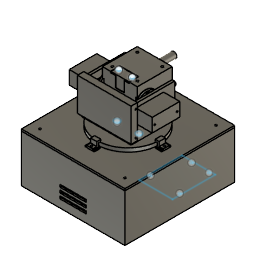
carro_armato_assieme_completo_modificabile_v5_cinematica_stepper_servo_M2_5 (Autodesk Fusion 360 design; units mm, degrees)
part number: 2026-07-14-04-41-23-405
part number: 2026-07-14-04-41-23-631
part number: 2026-07-14-04-41-23-666
part number: 2026-07-14-04-41-25-878
part number: 2026-07-14-04-41-28-136
part number: 2026-07-14-04-41-28-298
part number: 2026-07-14-04-41-30-257
part number: 2026-07-14-04-41-52-420
part number: 2026-07-14-04-41-53-406
part number: 2026-07-14-04-41-55-252
part number: 2026-07-14-04-41-56-766
part number: 2026-07-14-04-42-07-757
part number: 2026-07-14-04-42-11-829
part number: 2026-07-14-04-42-16-180
part number: 2026-07-14-04-42-20-616
part number: 2026-07-14-04-42-24-632
part number: 2026-07-14-04-43-20-199
part number: 2026-07-14-04-43-28-088
part number: 2026-07-14-04-43-36-335
part number: 2026-07-14-04-44-01-058
part number: 2026-07-14-04-44-07-569
part number: 2026-07-14-04-44-14-384
part number: 2026-07-14-04-44-23-421
part number: 2026-07-14-04-44-35-084
part number: 2026-07-14-04-44-58-859
part number: 2026-07-14-04-45-33-050
part number: 2026-07-14-04-45-52-643
part number: 2026-07-14-04-46-12-584
part number: 2026-07-14-04-47-47-358
Autodesk Fusion 360 part; units mm, degrees
(part 1 of 4)
sketch "Schizzo1" plane through (0, 0, 0) normal (0, 0, 1) x (1, 0, 0) in component "01_Piano_inferiore_colonnine_M3_supporto_batteria_integrato"
  line L0 (-80, -85) -> (80, -85)
  line L1 (80, -85) -> (80, 85)
  line L2 (80, 85) -> (-80, 85)
  line L3 (-80, 85) -> (-80, -85)
extrude "Estrusione_Piano_inferiore" add sketch "Schizzo1" along normal blind 3 makes body 1 in component "01_Piano_inferiore_colonnine_M3_supporto_batteria_integrato"
ref_plane "Piano di lavoro1" through (0, 0, 43) normal (0, 0, 1) x (1, 0, 0) in component "02_Piano_superiore"
sketch "Schizzo1 (2)" plane through (0, 0, 43) normal (0, 0, 1) x (1, 0, 0) in component "02_Piano_superiore"
  line L0 (-80, -85) -> (80, -85)
  line L1 (80, -85) -> (80, 85)
  line L2 (80, 85) -> (-80, 85)
  line L3 (-80, 85) -> (-80, -85)
extrude "Estrusione_Piano_superiore" add sketch "Schizzo1 (2)" along normal blind 3 separate body makes body 2 in component "02_Piano_superiore"
ref_plane "Piano di lavoro1" through (0, 0, 3) normal (0, 0, 1) x (1, 0, 0) in component "01_Piano_inferiore_colonnine_M3_supporto_batteria_integrato"
ref_plane "Piano di lavoro2" through (0, 0, 40.4) normal (0, 0, 1) x (1, 0, 0) in component "01_Piano_inferiore_colonnine_M3_supporto_batteria_integrato"
sketch "Schizzo2" plane through (0, 0, 0) normal (0, 0, 1) x (1, 0, 0) in component "01_Piano_inferiore_colonnine_M3_supporto_batteria_integrato"
  line L0 (-5, -77.5) -> (5, -77.5)
  line L1 (5, -77.5) -> (5, -72.5)
  line L2 (5, -72.5) -> (-5, -72.5)
  line L3 (-5, -72.5) -> (-5, -77.5)
extrude "Asola_fascetta_01" cut sketch "Schizzo2" along normal blind 3 bodies 1 in component "01_Piano_inferiore_colonnine_M3_supporto_batteria_integrato"
sketch "Schizzo3" plane through (0, 0, 0) normal (0, 0, 1) x (1, 0, 0) in component "01_Piano_inferiore_colonnine_M3_supporto_batteria_integrato"
  line L0 (-5, -62.5) -> (5, -62.5)
  line L1 (5, -62.5) -> (5, -57.5)
  line L2 (5, -57.5) -> (-5, -57.5)
  line L3 (-5, -57.5) -> (-5, -62.5)
extrude "Asola_fascetta_02" cut sketch "Schizzo3" along normal blind 3 bodies 1 in component "01_Piano_inferiore_colonnine_M3_supporto_batteria_integrato"
sketch "Schizzo4" plane through (0, 0, 0) normal (0, 0, 1) x (1, 0, 0) in component "01_Piano_inferiore_colonnine_M3_supporto_batteria_integrato"
  line L0 (-5, -12.5) -> (5, -12.5)
  line L1 (5, -12.5) -> (5, -7.5)
  line L2 (5, -7.5) -> (-5, -7.5)
  line L3 (-5, -7.5) -> (-5, -12.5)
extrude "Asola_fascetta_03" cut sketch "Schizzo4" along normal blind 3 bodies 1 in component "01_Piano_inferiore_colonnine_M3_supporto_batteria_integrato"
sketch "Schizzo5" plane through (0, 0, 0) normal (0, 0, 1) x (1, 0, 0) in component "01_Piano_inferiore_colonnine_M3_supporto_batteria_integrato"
  line L0 (-5, 2.5) -> (5, 2.5)
  line L1 (5, 2.5) -> (5, 7.5)
  line L2 (5, 7.5) -> (-5, 7.5)
  line L3 (-5, 7.5) -> (-5, 2.5)
extrude "Asola_fascetta_04" cut sketch "Schizzo5" along normal blind 3 bodies 1 in component "01_Piano_inferiore_colonnine_M3_supporto_batteria_integrato"
sketch "Schizzo6" plane through (0, 0, 0) normal (0, 0, 1) x (1, 0, 0) in component "01_Piano_inferiore_colonnine_M3_supporto_batteria_integrato"
  line L0 (-5.5, 20) -> (4.5, 20)
  line L1 (4.5, 20) -> (4.5, 30)
  line L2 (4.5, 30) -> (-5.5, 30)
  line L3 (-5.5, 30) -> (-5.5, 20)
extrude "Foro_servizio_10x10_vicino_Arduino" cut sketch "Schizzo6" along normal blind 3 bodies 1 in component "01_Piano_inferiore_colonnine_M3_supporto_batteria_integrato"
sketch "Schizzo2 (2)" plane through (0, 0, 43) normal (0, 0, 1) x (1, 0, 0) in component "02_Piano_superiore"
  circle A0 centre (-68, -73) radius 1.6
extrude "Foro_M3_superiore_01" cut sketch "Schizzo2 (2)" along normal blind 3 bodies 2 in component "02_Piano_superiore"
sketch "Schizzo7" plane through (0, 0, 3) normal (0, 0, 1) x (1, 0, 0) in component "01_Piano_inferiore_colonnine_M3_supporto_batteria_integrato"
  circle A0 centre (-68, -73) radius 5
extrude "Estrusione_Colonnina_M3_01" add sketch "Schizzo7" along normal blind 40 bodies 1 in component "01_Piano_inferiore_colonnine_M3_supporto_batteria_integrato"
sketch "Schizzo8" plane through (0, 0, 0) normal (0, 0, 1) x (1, 0, 0) in component "01_Piano_inferiore_colonnine_M3_supporto_batteria_integrato"
  circle A0 centre (-68, -73) radius 1.6
extrude "Foro_passante_M3_colonnina_01" cut sketch "Schizzo8" along normal blind 43 bodies 1 in component "01_Piano_inferiore_colonnine_M3_supporto_batteria_integrato"
sketch "Schizzo9" plane through (0, 0, 40.4) normal (0, 0, 1) x (1, 0, 0) in component "01_Piano_inferiore_colonnine_M3_supporto_batteria_integrato"
  line L0 (-65.1, -71.3257) -> (-68, -69.6514)
  line L1 (-68, -69.6514) -> (-70.9, -71.3257)
  line L2 (-70.9, -71.3257) -> (-70.9, -74.6743)
  line L3 (-70.9, -74.6743) -> (-68, -76.3486)
  line L4 (-68, -76.3486) -> (-65.1, -74.6743)
  line L5 (-65.1, -74.6743) -> (-65.1, -71.3257)
extrude "Sede_dado_M3_01" cut sketch "Schizzo9" along normal blind 2.6 bodies 1 in component "01_Piano_inferiore_colonnine_M3_supporto_batteria_integrato"
sketch "Schizzo3 (2)" plane through (0, 0, 43) normal (0, 0, 1) x (1, 0, 0) in component "02_Piano_superiore"
  circle A0 centre (68, -73) radius 1.6
extrude "Foro_M3_superiore_02" cut sketch "Schizzo3 (2)" along normal blind 3 bodies 2 in component "02_Piano_superiore"
sketch "Schizzo10" plane through (0, 0, 3) normal (0, 0, 1) x (1, 0, 0) in component "01_Piano_inferiore_colonnine_M3_supporto_batteria_integrato"
  circle A0 centre (68, -73) radius 5
extrude "Estrusione_Colonnina_M3_02" add sketch "Schizzo10" along normal blind 40 bodies 1 in component "01_Piano_inferiore_colonnine_M3_supporto_batteria_integrato"
sketch "Schizzo11" plane through (0, 0, 0) normal (0, 0, 1) x (1, 0, 0) in component "01_Piano_inferiore_colonnine_M3_supporto_batteria_integrato"
  circle A0 centre (68, -73) radius 1.6
extrude "Foro_passante_M3_colonnina_02" cut sketch "Schizzo11" along normal blind 43 bodies 1 in component "01_Piano_inferiore_colonnine_M3_supporto_batteria_integrato"
sketch "Schizzo12" plane through (0, 0, 40.4) normal (0, 0, 1) x (1, 0, 0) in component "01_Piano_inferiore_colonnine_M3_supporto_batteria_integrato"
  line L0 (70.9, -71.3257) -> (68, -69.6514)
  line L1 (68, -69.6514) -> (65.1, -71.3257)
  line L2 (65.1, -71.3257) -> (65.1, -74.6743)
  line L3 (65.1, -74.6743) -> (68, -76.3486)
  line L4 (68, -76.3486) -> (70.9, -74.6743)
  line L5 (70.9, -74.6743) -> (70.9, -71.3257)
extrude "Sede_dado_M3_02" cut sketch "Schizzo12" along normal blind 2.6 bodies 1 in component "01_Piano_inferiore_colonnine_M3_supporto_batteria_integrato"
sketch "Schizzo4 (2)" plane through (0, 0, 43) normal (0, 0, 1) x (1, 0, 0) in component "02_Piano_superiore"
  circle A0 centre (68, 73) radius 1.6
extrude "Foro_M3_superiore_03" cut sketch "Schizzo4 (2)" along normal blind 3 bodies 2 in component "02_Piano_superiore"
sketch "Schizzo13" plane through (0, 0, 3) normal (0, 0, 1) x (1, 0, 0) in component "01_Piano_inferiore_colonnine_M3_supporto_batteria_integrato"
  circle A0 centre (68, 73) radius 5
extrude "Estrusione_Colonnina_M3_03" add sketch "Schizzo13" along normal blind 40 bodies 1 in component "01_Piano_inferiore_colonnine_M3_supporto_batteria_integrato"
sketch "Schizzo14" plane through (0, 0, 0) normal (0, 0, 1) x (1, 0, 0) in component "01_Piano_inferiore_colonnine_M3_supporto_batteria_integrato"
  circle A0 centre (68, 73) radius 1.6
extrude "Foro_passante_M3_colonnina_03" cut sketch "Schizzo14" along normal blind 43 bodies 1 in component "01_Piano_inferiore_colonnine_M3_supporto_batteria_integrato"
sketch "Schizzo15" plane through (0, 0, 40.4) normal (0, 0, 1) x (1, 0, 0) in component "01_Piano_inferiore_colonnine_M3_supporto_batteria_integrato"
  line L0 (70.9, 74.6743) -> (68, 76.3486)
  line L1 (68, 76.3486) -> (65.1, 74.6743)
  line L2 (65.1, 74.6743) -> (65.1, 71.3257)
  line L3 (65.1, 71.3257) -> (68, 69.6514)
  line L4 (68, 69.6514) -> (70.9, 71.3257)
  line L5 (70.9, 71.3257) -> (70.9, 74.6743)
extrude "Sede_dado_M3_03" cut sketch "Schizzo15" along normal blind 2.6 bodies 1 in component "01_Piano_inferiore_colonnine_M3_supporto_batteria_integrato"
sketch "Schizzo5 (2)" plane through (0, 0, 43) normal (0, 0, 1) x (1, 0, 0) in component "02_Piano_superiore"
  circle A0 centre (-68, 73) radius 1.6
extrude "Foro_M3_superiore_04" cut sketch "Schizzo5 (2)" along normal blind 3 bodies 2 in component "02_Piano_superiore"
sketch "Schizzo16" plane through (0, 0, 3) normal (0, 0, 1) x (1, 0, 0) in component "01_Piano_inferiore_colonnine_M3_supporto_batteria_integrato"
  circle A0 centre (-68, 73) radius 5
extrude "Estrusione_Colonnina_M3_04" add sketch "Schizzo16" along normal blind 40 bodies 1 in component "01_Piano_inferiore_colonnine_M3_supporto_batteria_integrato"
sketch "Schizzo17" plane through (0, 0, 0) normal (0, 0, 1) x (1, 0, 0) in component "01_Piano_inferiore_colonnine_M3_supporto_batteria_integrato"
  circle A0 centre (-68, 73) radius 1.6
extrude "Foro_passante_M3_colonnina_04" cut sketch "Schizzo17" along normal blind 43 bodies 1 in component "01_Piano_inferiore_colonnine_M3_supporto_batteria_integrato"
sketch "Schizzo18" plane through (0, 0, 40.4) normal (0, 0, 1) x (1, 0, 0) in component "01_Piano_inferiore_colonnine_M3_supporto_batteria_integrato"
  line L0 (-65.1, 74.6743) -> (-68, 76.3486)
  line L1 (-68, 76.3486) -> (-70.9, 74.6743)
  line L2 (-70.9, 74.6743) -> (-70.9, 71.3257)
  line L3 (-70.9, 71.3257) -> (-68, 69.6514)
  line L4 (-68, 69.6514) -> (-65.1, 71.3257)
  line L5 (-65.1, 71.3257) -> (-65.1, 74.6743)
extrude "Sede_dado_M3_04" cut sketch "Schizzo18" along normal blind 2.6 bodies 1 in component "01_Piano_inferiore_colonnine_M3_supporto_batteria_integrato"
sketch "Schizzo6 (2)" plane through (0, 0, 43) normal (0, 0, 1) x (1, 0, 0) in component "02_Piano_superiore"
  line L0 (20.83, 33.21) -> (45.83, 33.21)
  line L1 (45.83, 33.21) -> (45.83, 58.21)
  line L2 (45.83, 58.21) -> (20.83, 58.21)
  line L3 (20.83, 58.21) -> (20.83, 33.21)
extrude "Apertura_Arduino_25x25_D2_D7_S1_S8" cut sketch "Schizzo6 (2)" along normal blind 3 bodies 2 in component "02_Piano_superiore"
sketch "Schizzo7 (2)" plane through (0, 0, 43) normal (0, 0, 1) x (1, 0, 0) in component "02_Piano_superiore"
  line L0 (-69, -45) -> (-36, -45)
  line L1 (-36, -45) -> (-36, 15)
  line L2 (-36, 15) -> (-69, 15)
  line L3 (-69, 15) -> (-69, -45)
extrude "Apertura_pacco_batteria_PCB_cannone_60x33" cut sketch "Schizzo7 (2)" along normal blind 3 bodies 2 in component "02_Piano_superiore"
sketch "Schizzo8 (2)" plane through (0, 0, 43) normal (0, 0, 1) x (1, 0, 0) in component "02_Piano_superiore"
  circle A0 centre (0, -79.5) radius 1.35
extrude "Foro_M2_5_guscio_inferiore_01_south" cut sketch "Schizzo8 (2)" along normal blind 3 bodies 2 in component "02_Piano_superiore"
sketch "Schizzo9 (2)" plane through (0, 0, 43) normal (0, 0, 1) x (1, 0, 0) in component "02_Piano_superiore"
  circle A0 centre (0, 79.5) radius 1.35
extrude "Foro_M2_5_guscio_inferiore_02_north" cut sketch "Schizzo9 (2)" along normal blind 3 bodies 2 in component "02_Piano_superiore"
sketch "Schizzo10 (2)" plane through (0, 0, 43) normal (0, 0, 1) x (1, 0, 0) in component "02_Piano_superiore"
  circle A0 centre (74.5, 45) radius 1.35
extrude "Foro_M2_5_guscio_inferiore_03_east" cut sketch "Schizzo10 (2)" along normal blind 3 bodies 2 in component "02_Piano_superiore"
sketch "Schizzo11 (2)" plane through (0, 0, 43) normal (0, 0, 1) x (1, 0, 0) in component "02_Piano_superiore"
  circle A0 centre (-74.5, 45) radius 1.35
extrude "Foro_M2_5_guscio_inferiore_04_west" cut sketch "Schizzo11 (2)" along normal blind 3 bodies 2 in component "02_Piano_superiore"
ref_plane "Piano di lavoro3" through (0, 0, 3) normal (0, 0, 1) x (1, 0, 0) in component "01_Piano_inferiore_colonnine_M3_supporto_batteria_integrato"
sketch "Schizzo19" plane through (0, 0, 3) normal (0, 0, 1) x (1, 0, 0) in component "01_Piano_inferiore_colonnine_M3_supporto_batteria_integrato"
  line L0 (-75, -65) -> (-72.5, -65)
  line L1 (-72.5, -65) -> (-72.5, 35)
  line L2 (-72.5, 35) -> (-75, 35)
  line L3 (-75, 35) -> (-75, -65)
extrude "Estrusione_Parete_lunga_Ovest" add sketch "Schizzo19" along normal blind 17 bodies 1 in component "01_Piano_inferiore_colonnine_M3_supporto_batteria_integrato"
sketch "Schizzo20" plane through (0, 0, 3) normal (0, 0, 1) x (1, 0, 0) in component "01_Piano_inferiore_colonnine_M3_supporto_batteria_integrato"
  line L0 (-32.5, -65) -> (-30, -65)
  line L1 (-30, -65) -> (-30, 35)
  line L2 (-30, 35) -> (-32.5, 35)
  line L3 (-32.5, 35) -> (-32.5, -65)
extrude "Estrusione_Parete_lunga_Est" add sketch "Schizzo20" along normal blind 17 bodies 1 in component "01_Piano_inferiore_colonnine_M3_supporto_batteria_integrato"
sketch "Schizzo21" plane through (0, 0, 3) normal (0, 0, 1) x (1, 0, 0) in component "01_Piano_inferiore_colonnine_M3_supporto_batteria_integrato"
  line L0 (-75, -65) -> (-30, -65)
  line L1 (-30, -65) -> (-30, -60)
  line L2 (-30, -60) -> (-75, -60)
  line L3 (-75, -60) -> (-75, -65)
extrude "Estrusione_Parete_corta_chiusa" add sketch "Schizzo21" along normal blind 17 bodies 1 in component "01_Piano_inferiore_colonnine_M3_supporto_batteria_integrato"
sketch "Schizzo22" plane through (0, 0, 3) normal (0, 0, 1) x (1, 0, 0) in component "01_Piano_inferiore_colonnine_M3_supporto_batteria_integrato"
  line L0 (-32.6, -60) -> (-29.9, -60)
  line L1 (-29.9, -60) -> (-29.9, -50)
  line L2 (-29.9, -50) -> (-32.6, -50)
  line L3 (-32.6, -50) -> (-32.6, -60)
extrude "Apertura_cavi_parete_lunga_Est" cut sketch "Schizzo22" along normal blind 17 bodies 1 in component "01_Piano_inferiore_colonnine_M3_supporto_batteria_integrato"
sketch "Schizzo1 (3)" plane through (0, 0, 0) normal (0, 0, 1) x (1, 0, 0) in component "03_Guscio_laterale_continuo_carro"
  line L0 (-83, -88) -> (-80.5, -88)
  line L1 (-80.5, -88) -> (-80.5, 88)
  line L2 (-80.5, 88) -> (-83, 88)
  line L3 (-83, 88) -> (-83, -88)
extrude "Estrusione_Parete_guscio_Ovest" add sketch "Schizzo1 (3)" along normal blind 76 separate body makes body 3 in component "03_Guscio_laterale_continuo_carro"
sketch "Schizzo2 (3)" plane through (0, 0, 0) normal (0, 0, 1) x (1, 0, 0) in component "03_Guscio_laterale_continuo_carro"
  line L0 (-83, -88) -> (83, -88)
  line L1 (83, -88) -> (83, -85.5)
  line L2 (83, -85.5) -> (-83, -85.5)
  line L3 (-83, -85.5) -> (-83, -88)
extrude "Estrusione_Parete_guscio_Sud" add sketch "Schizzo2 (3)" along normal blind 76 bodies 3 in component "03_Guscio_laterale_continuo_carro"
sketch "Schizzo3 (3)" plane through (0, 0, 0) normal (0, 0, 1) x (1, 0, 0) in component "03_Guscio_laterale_continuo_carro"
  line L0 (80.5, -88) -> (83, -88)
  line L1 (83, -88) -> (83, 88)
  line L2 (83, 88) -> (80.5, 88)
  line L3 (80.5, 88) -> (80.5, -88)
extrude "Estrusione_Parete_guscio_Est" add sketch "Schizzo3 (3)" along normal blind 76 bodies 3 in component "03_Guscio_laterale_continuo_carro"
sketch "Schizzo4 (3)" plane through (0, 0, 0) normal (0, 0, 1) x (1, 0, 0) in component "03_Guscio_laterale_continuo_carro"
  line L0 (-83, 85.5) -> (83, 85.5)
  line L1 (83, 85.5) -> (83, 88)
  line L2 (83, 88) -> (-83, 88)
  line L3 (-83, 88) -> (-83, 85.5)
extrude "Estrusione_Parete_guscio_Nord" add sketch "Schizzo4 (3)" along normal blind 76 bodies 3 in component "03_Guscio_laterale_continuo_carro"
ref_plane "Piano di lavoro1" through (0, -88, 0) normal (0, 1, 0) x (0, 0, 1) in component "03_Guscio_laterale_continuo_carro"
sketch "Schizzo5 (3)" plane through (0, -88, 0) normal (0, 1, 0) x (1, 0, 0) in component "03_Guscio_laterale_continuo_carro"
  line L0 (-21, -13) -> (21, -13)
  line L1 (21, -13) -> (21, -17)
  line L2 (21, -17) -> (-21, -17)
  line L3 (-21, -17) -> (-21, -13)
extrude "Griglia_Posteriore_Sud_01" cut sketch "Schizzo5 (3)" along normal blind 2.7 bodies 3 in component "03_Guscio_laterale_continuo_carro"
ref_plane "Piano di lavoro2" through (0, -88, 0) normal (0, 1, 0) x (0, 0, 1) in component "03_Guscio_laterale_continuo_carro"
sketch "Schizzo6 (3)" plane through (0, -88, 0) normal (0, 1, 0) x (1, 0, 0) in component "03_Guscio_laterale_continuo_carro"
  line L0 (-21, -21) -> (21, -21)
  line L1 (21, -21) -> (21, -25)
  line L2 (21, -25) -> (-21, -25)
  line L3 (-21, -25) -> (-21, -21)
extrude "Griglia_Posteriore_Sud_02" cut sketch "Schizzo6 (3)" along normal blind 2.7 bodies 3 in component "03_Guscio_laterale_continuo_carro"
ref_plane "Piano di lavoro3" through (0, -88, 0) normal (0, 1, 0) x (0, 0, 1) in component "03_Guscio_laterale_continuo_carro"
sketch "Schizzo7 (3)" plane through (0, -88, 0) normal (0, 1, 0) x (1, 0, 0) in component "03_Guscio_laterale_continuo_carro"
  line L0 (-21, -29) -> (21, -29)
  line L1 (21, -29) -> (21, -33)
  line L2 (21, -33) -> (-21, -33)
  line L3 (-21, -33) -> (-21, -29)
extrude "Griglia_Posteriore_Sud_03" cut sketch "Schizzo7 (3)" along normal blind 2.7 bodies 3 in component "03_Guscio_laterale_continuo_carro"
ref_plane "Piano di lavoro4" through (0, 85.5, 0) normal (0, 1, 0) x (0, 0, 1) in component "03_Guscio_laterale_continuo_carro"
sketch "Schizzo8 (3)" plane through (0, 85.5, 0) normal (0, 1, 0) x (1, 0, 0) in component "03_Guscio_laterale_continuo_carro"
  line L0 (-21, -13) -> (21, -13)
  line L1 (21, -13) -> (21, -17)
  line L2 (21, -17) -> (-21, -17)
  line L3 (-21, -17) -> (-21, -13)
extrude "Griglia_Anteriore_Nord_01" cut sketch "Schizzo8 (3)" along normal blind 2.7 bodies 3 in component "03_Guscio_laterale_continuo_carro"
ref_plane "Piano di lavoro5" through (0, 85.5, 0) normal (0, 1, 0) x (0, 0, 1) in component "03_Guscio_laterale_continuo_carro"
sketch "Schizzo9 (3)" plane through (0, 85.5, 0) normal (0, 1, 0) x (1, 0, 0) in component "03_Guscio_laterale_continuo_carro"
  line L0 (-21, -21) -> (21, -21)
  line L1 (21, -21) -> (21, -25)
  line L2 (21, -25) -> (-21, -25)
  line L3 (-21, -25) -> (-21, -21)
extrude "Griglia_Anteriore_Nord_02" cut sketch "Schizzo9 (3)" along normal blind 2.7 bodies 3 in component "03_Guscio_laterale_continuo_carro"
ref_plane "Piano di lavoro6" through (0, 85.5, 0) normal (0, 1, 0) x (0, 0, 1) in component "03_Guscio_laterale_continuo_carro"
sketch "Schizzo10 (3)" plane through (0, 85.5, 0) normal (0, 1, 0) x (1, 0, 0) in component "03_Guscio_laterale_continuo_carro"
  line L0 (-21, -29) -> (21, -29)
  line L1 (21, -29) -> (21, -33)
  line L2 (21, -33) -> (-21, -33)
  line L3 (-21, -33) -> (-21, -29)
extrude "Griglia_Anteriore_Nord_03" cut sketch "Schizzo10 (3)" along normal blind 2.7 bodies 3 in component "03_Guscio_laterale_continuo_carro"
ref_plane "Piano di lavoro7" through (0, 0, 38) normal (0, 0, 1) x (1, 0, 0) in component "03_Guscio_laterale_continuo_carro"
sketch "Schizzo11 (3)" plane through (0, 0, 38) normal (0, 0, 1) x (1, 0, 0) in component "03_Guscio_laterale_continuo_carro"
  line L0 (-7, -86) -> (7, -86)
  line L1 (7, -86) -> (7, -73)
  line L2 (7, -73) -> (-7, -73)
  line L3 (-7, -73) -> (-7, -86)
extrude "Estrusione_Linguetta_M2_5_01_south" add sketch "Schizzo11 (3)" along normal blind 5 bodies 3 in component "03_Guscio_laterale_continuo_carro"
sketch "Schizzo12 (2)" plane through (0, 0, 38) normal (0, 0, 1) x (1, 0, 0) in component "03_Guscio_laterale_continuo_carro"
  circle A0 centre (0, -79.5) radius 1.1
extrude "Preforo_M2_5_guscio_01_south" cut sketch "Schizzo12 (2)" along normal blind 5 bodies 3 in component "03_Guscio_laterale_continuo_carro"
sketch "Schizzo13 (2)" plane through (0, 0, 38) normal (0, 0, 1) x (1, 0, 0) in component "03_Guscio_laterale_continuo_carro"
  line L0 (-7, 73) -> (7, 73)
  line L1 (7, 73) -> (7, 86)
  line L2 (7, 86) -> (-7, 86)
  line L3 (-7, 86) -> (-7, 73)
extrude "Estrusione_Linguetta_M2_5_02_north" add sketch "Schizzo13 (2)" along normal blind 5 bodies 3 in component "03_Guscio_laterale_continuo_carro"
sketch "Schizzo14 (2)" plane through (0, 0, 38) normal (0, 0, 1) x (1, 0, 0) in component "03_Guscio_laterale_continuo_carro"
  circle A0 centre (0, 79.5) radius 1.1
extrude "Preforo_M2_5_guscio_02_north" cut sketch "Schizzo14 (2)" along normal blind 5 bodies 3 in component "03_Guscio_laterale_continuo_carro"
sketch "Schizzo15 (2)" plane through (0, 0, 38) normal (0, 0, 1) x (1, 0, 0) in component "03_Guscio_laterale_continuo_carro"
  line L0 (68, 38) -> (81, 38)
  line L1 (81, 38) -> (81, 52)
  line L2 (81, 52) -> (68, 52)
  line L3 (68, 52) -> (68, 38)
extrude "Estrusione_Linguetta_M2_5_03_east" add sketch "Schizzo15 (2)" along normal blind 5 bodies 3 in component "03_Guscio_laterale_continuo_carro"
sketch "Schizzo16 (2)" plane through (0, 0, 38) normal (0, 0, 1) x (1, 0, 0) in component "03_Guscio_laterale_continuo_carro"
  circle A0 centre (74.5, 45) radius 1.1
extrude "Preforo_M2_5_guscio_03_east" cut sketch "Schizzo16 (2)" along normal blind 5 bodies 3 in component "03_Guscio_laterale_continuo_carro"
sketch "Schizzo17 (2)" plane through (0, 0, 38) normal (0, 0, 1) x (1, 0, 0) in component "03_Guscio_laterale_continuo_carro"
  line L0 (-81, 38) -> (-68, 38)
  line L1 (-68, 38) -> (-68, 52)
  line L2 (-68, 52) -> (-81, 52)
  line L3 (-81, 52) -> (-81, 38)
extrude "Estrusione_Linguetta_M2_5_04_west" add sketch "Schizzo17 (2)" along normal blind 5 bodies 3 in component "03_Guscio_laterale_continuo_carro"
sketch "Schizzo18 (2)" plane through (0, 0, 38) normal (0, 0, 1) x (1, 0, 0) in component "03_Guscio_laterale_continuo_carro"
  circle A0 centre (-74.5, 45) radius 1.1
extrude "Preforo_M2_5_guscio_04_west" cut sketch "Schizzo18 (2)" along normal blind 5 bodies 3 in component "03_Guscio_laterale_continuo_carro"
sketch "Schizzo1 (4)" plane through (0, 0, 0) normal (0, 0, 1) x (1, 0, 0) in component "05_Arduino_UNO_R4_WiFi_RIFERIMENTO_XY_quota_Z_da_definire"
  line L0 (-26.67, -34.29) -> (26.67, -34.29)
  line L1 (26.67, -34.29) -> (26.67, 34.29)
  line L2 (26.67, 34.29) -> (-26.67, 34.29)
  line L3 (-26.67, 34.29) -> (-26.67, -34.29)
  circle A0 centre (24.13, -20.32) radius 1.6
  circle A1 centre (-24.13, -19.05) radius 1.6
  circle A2 centre (19.05, 31.75) radius 1.6
  circle A3 centre (-8.89, 31.75) radius 1.6
ref_plane "Piano di lavoro1" through (0, 0, 30) normal (0, 0, 1) x (1, 0, 0) in component "01_Tetto_elettronica_removibile"
sketch "Schizzo1 (5)" plane through (0, 0, 30) normal (0, 0, 1) x (1, 0, 0) in component "01_Tetto_elettronica_removibile"
  line L0 (-83, -88) -> (83, -88)
  line L1 (83, -88) -> (83, 88)
  line L2 (83, 88) -> (-83, 88)
  line L3 (-83, 88) -> (-83, -88)
extrude "Estrusione_Tetto_coperchio" add sketch "Schizzo1 (5)" along normal blind 3 separate body makes body 4 in component "01_Tetto_elettronica_removibile"
sketch "Schizzo2 (4)" plane through (0, 0, 0) normal (0, 0, 1) x (1, 0, 0) in component "01_Tetto_elettronica_removibile"
  circle A0 centre (-68, -73) radius 5
extrude "Estrusione_Boss_verticale_M3_coperchio_01" add sketch "Schizzo2 (4)" along normal blind 33 bodies 4 in component "01_Tetto_elettronica_removibile"
sketch "Schizzo3 (4)" plane through (0, 0, 0) normal (0, 0, 1) x (1, 0, 0) in component "01_Tetto_elettronica_removibile"
  circle A0 centre (-68, -73) radius 1.6
extrude "Foro_M3_accessibile_dal_tetto_01" cut sketch "Schizzo3 (4)" along normal blind 33 bodies 4 in component "01_Tetto_elettronica_removibile"
sketch "Schizzo4 (4)" plane through (0, 0, 0) normal (0, 0, 1) x (1, 0, 0) in component "01_Tetto_elettronica_removibile"
  circle A0 centre (68, -73) radius 5
extrude "Estrusione_Boss_verticale_M3_coperchio_02" add sketch "Schizzo4 (4)" along normal blind 33 bodies 4 in component "01_Tetto_elettronica_removibile"
sketch "Schizzo5 (4)" plane through (0, 0, 0) normal (0, 0, 1) x (1, 0, 0) in component "01_Tetto_elettronica_removibile"
  circle A0 centre (68, -73) radius 1.6
extrude "Foro_M3_accessibile_dal_tetto_02" cut sketch "Schizzo5 (4)" along normal blind 33 bodies 4 in component "01_Tetto_elettronica_removibile"
sketch "Schizzo6 (4)" plane through (0, 0, 0) normal (0, 0, 1) x (1, 0, 0) in component "01_Tetto_elettronica_removibile"
  circle A0 centre (-68, 73) radius 5
extrude "Estrusione_Boss_verticale_M3_coperchio_03" add sketch "Schizzo6 (4)" along normal blind 33 bodies 4 in component "01_Tetto_elettronica_removibile"
sketch "Schizzo7 (4)" plane through (0, 0, 0) normal (0, 0, 1) x (1, 0, 0) in component "01_Tetto_elettronica_removibile"
  circle A0 centre (-68, 73) radius 1.6
extrude "Foro_M3_accessibile_dal_tetto_03" cut sketch "Schizzo7 (4)" along normal blind 33 bodies 4 in component "01_Tetto_elettronica_removibile"
sketch "Schizzo8 (4)" plane through (0, 0, 0) normal (0, 0, 1) x (1, 0, 0) in component "01_Tetto_elettronica_removibile"
  circle A0 centre (68, 73) radius 5
extrude "Estrusione_Boss_verticale_M3_coperchio_04" add sketch "Schizzo8 (4)" along normal blind 33 bodies 4 in component "01_Tetto_elettronica_removibile"
sketch "Schizzo9 (4)" plane through (0, 0, 0) normal (0, 0, 1) x (1, 0, 0) in component "01_Tetto_elettronica_removibile"
  circle A0 centre (68, 73) radius 1.6
extrude "Foro_M3_accessibile_dal_tetto_04" cut sketch "Schizzo9 (4)" along normal blind 33 bodies 4 in component "01_Tetto_elettronica_removibile"
ref_plane "Piano di lavoro2" through (0, 0, 30) normal (0, 0, 1) x (1, 0, 0) in component "01_Tetto_elettronica_removibile"
ref_plane "Piano di lavoro3" through (0, 0, 33) normal (0, 0, 1) x (1, 0, 0) in component "01_Tetto_elettronica_removibile"
ref_plane "Piano di lavoro4" through (0, 0, 30.9) normal (0, 0, 1) x (1, 0, 0) in component "01_Tetto_elettronica_removibile"
sketch "Schizzo10 (4)" plane through (0, 0, 30) normal (0, 0, 1) x (1, 0, 0) in component "01_Tetto_elettronica_removibile"
  circle A0 centre (0, 0) radius 4
extrude "Passaggio_albero_stepper" cut sketch "Schizzo10 (4)" along normal blind 3 bodies 4 in component "01_Tetto_elettronica_removibile"
sketch "Schizzo11 (4)" plane through (0, 0, 30) normal (0, 0, 1) x (1, 0, 0) in component "01_Tetto_elettronica_removibile"
  circle A0 centre (-17.5, 0) radius 2.1
extrude "Foro_stepper_Ovest" cut sketch "Schizzo11 (4)" along normal blind 3 bodies 4 in component "01_Tetto_elettronica_removibile"
sketch "Schizzo12 (3)" plane through (0, 0, 30.9) normal (0, 0, 1) x (1, 0, 0) in component "01_Tetto_elettronica_removibile"
  circle A0 centre (-17.5, 0) radius 2.1
sketch "Schizzo13 (3)" plane through (0, 0, 33) normal (0, 0, 1) x (1, 0, 0) in component "01_Tetto_elettronica_removibile"
  circle A0 centre (-17.5, 0) radius 4.2
loft "Svasatura_90_gradi_stepper_Ovest" cut profiles "Schizzo12 (3)", "Schizzo13 (3)" section 1 section 2 bodies 4 in component "01_Tetto_elettronica_removibile"
sketch "Schizzo14 (3)" plane through (0, 0, 30) normal (0, 0, 1) x (1, 0, 0) in component "01_Tetto_elettronica_removibile"
  circle A0 centre (17.5, 0) radius 2.1
extrude "Foro_stepper_Est" cut sketch "Schizzo14 (3)" along normal blind 3 bodies 4 in component "01_Tetto_elettronica_removibile"
sketch "Schizzo15 (3)" plane through (0, 0, 30.9) normal (0, 0, 1) x (1, 0, 0) in component "01_Tetto_elettronica_removibile"
  circle A0 centre (17.5, 0) radius 2.1
sketch "Schizzo16 (3)" plane through (0, 0, 33) normal (0, 0, 1) x (1, 0, 0) in component "01_Tetto_elettronica_removibile"
  circle A0 centre (17.5, 0) radius 4.2
loft "Svasatura_90_gradi_stepper_Est" cut profiles "Schizzo15 (3)", "Schizzo16 (3)" section 1 section 2 bodies 4 in component "01_Tetto_elettronica_removibile"
sketch "Schizzo17 (3)" plane through (0, 0, 30) normal (0, 0, 1) x (1, 0, 0) in component "01_Tetto_elettronica_removibile"
  circle A0 centre (58.5, 0) radius 1.6
extrude "Foro_M3_fermaglio_anti_sollevamento_Est" cut sketch "Schizzo17 (3)" along normal blind 3 bodies 4 in component "01_Tetto_elettronica_removibile"
sketch "Schizzo18 (3)" plane through (0, 0, 30) normal (0, 0, 1) x (1, 0, 0) in component "01_Tetto_elettronica_removibile"
  line L0 (61.4, 1.6743) -> (58.5, 3.3486)
  line L1 (58.5, 3.3486) -> (55.6, 1.6743)
  line L2 (55.6, 1.6743) -> (55.6, -1.6743)
  line L3 (55.6, -1.6743) -> (58.5, -3.3486)
  line L4 (58.5, -3.3486) -> (61.4, -1.6743)
  line L5 (61.4, -1.6743) -> (61.4, 1.6743)
extrude "Sede_dado_M3_fermaglio_Est" cut sketch "Schizzo18 (3)" along normal blind 2.6 bodies 4 in component "01_Tetto_elettronica_removibile"
sketch "Schizzo19 (2)" plane through (0, 0, 30) normal (0, 0, 1) x (1, 0, 0) in component "01_Tetto_elettronica_removibile"
  circle A0 centre (-58.5, 0) radius 1.6
extrude "Foro_M3_fermaglio_anti_sollevamento_Ovest" cut sketch "Schizzo19 (2)" along normal blind 3 bodies 4 in component "01_Tetto_elettronica_removibile"
sketch "Schizzo20 (2)" plane through (0, 0, 30) normal (0, 0, 1) x (1, 0, 0) in component "01_Tetto_elettronica_removibile"
  line L0 (-55.6, 1.6743) -> (-58.5, 3.3486)
  line L1 (-58.5, 3.3486) -> (-61.4, 1.6743)
  line L2 (-61.4, 1.6743) -> (-61.4, -1.6743)
  line L3 (-61.4, -1.6743) -> (-58.5, -3.3486)
  line L4 (-58.5, -3.3486) -> (-55.6, -1.6743)
  line L5 (-55.6, -1.6743) -> (-55.6, 1.6743)
extrude "Sede_dado_M3_fermaglio_Ovest" cut sketch "Schizzo20 (2)" along normal blind 2.6 bodies 4 in component "01_Tetto_elettronica_removibile"
sketch "Schizzo21 (2)" plane through (0, 0, 30) normal (0, 0, 1) x (1, 0, 0) in component "01_Tetto_elettronica_removibile"
  circle A0 centre (0, 58.5) radius 1.6
extrude "Foro_M3_fermaglio_anti_sollevamento_Nord" cut sketch "Schizzo21 (2)" along normal blind 3 bodies 4 in component "01_Tetto_elettronica_removibile"
sketch "Schizzo22 (2)" plane through (0, 0, 30) normal (0, 0, 1) x (1, 0, 0) in component "01_Tetto_elettronica_removibile"
  line L0 (2.9, 60.1743) -> (0, 61.8486)
  line L1 (0, 61.8486) -> (-2.9, 60.1743)
  line L2 (-2.9, 60.1743) -> (-2.9, 56.8257)
  line L3 (-2.9, 56.8257) -> (0, 55.1514)
  line L4 (0, 55.1514) -> (2.9, 56.8257)
  line L5 (2.9, 56.8257) -> (2.9, 60.1743)
extrude "Sede_dado_M3_fermaglio_Nord" cut sketch "Schizzo22 (2)" along normal blind 2.6 bodies 4 in component "01_Tetto_elettronica_removibile"
sketch "Schizzo23" plane through (0, 0, 30) normal (0, 0, 1) x (1, 0, 0) in component "01_Tetto_elettronica_removibile"
  circle A0 centre (0, -58.5) radius 1.6
extrude "Foro_M3_fermaglio_anti_sollevamento_Sud" cut sketch "Schizzo23" along normal blind 3 bodies 4 in component "01_Tetto_elettronica_removibile"
sketch "Schizzo24" plane through (0, 0, 30) normal (0, 0, 1) x (1, 0, 0) in component "01_Tetto_elettronica_removibile"
  line L0 (2.9, -56.8257) -> (0, -55.1514)
  line L1 (0, -55.1514) -> (-2.9, -56.8257)
  line L2 (-2.9, -56.8257) -> (-2.9, -60.1743)
  line L3 (-2.9, -60.1743) -> (0, -61.8486)
  line L4 (0, -61.8486) -> (2.9, -60.1743)
  line L5 (2.9, -60.1743) -> (2.9, -56.8257)
extrude "Sede_dado_M3_fermaglio_Sud" cut sketch "Schizzo24" along normal blind 2.6 bodies 4 in component "01_Tetto_elettronica_removibile"
ref_plane "Piano di lavoro5" through (0, 0, 22.8) normal (0, 0, 1) x (1, 0, 0) in component "01_Tetto_elettronica_removibile"
sketch "Schizzo25" plane through (0, 0, 22.8) normal (0, 0, 1) x (1, 0, 0) in component "01_Tetto_elettronica_removibile"
  circle A0 centre (0, 0) radius 23.5
  circle A1 centre (0, 0) radius 22
extrude "Estrusione_Parete_interna_liscia_canale_cavi" add sketch "Schizzo25" along normal blind 7.4 bodies 4 in component "01_Tetto_elettronica_removibile"
sketch "Schizzo26" plane through (0, 0, 22.8) normal (0, 0, 1) x (1, 0, 0) in component "01_Tetto_elettronica_removibile"
  circle A0 centre (0, 0) radius 34
  circle A1 centre (0, 0) radius 32.5
extrude "Estrusione_Parete_esterna_liscia_canale_cavi" add sketch "Schizzo26" along normal blind 7.4 bodies 4 in component "01_Tetto_elettronica_removibile"
ref_plane "Piano di lavoro6" through (0, 0, 20) normal (0, 0, 1) x (1, 0, 0) in component "01_Tetto_elettronica_removibile"
sketch "Schizzo27" plane through (0, 0, 20) normal (0, 0, 1) x (1, 0, 0) in component "01_Tetto_elettronica_removibile"
  circle A0 centre (0, 0) radius 40
  circle A1 centre (0, 0) radius 19
extrude "Estrusione_Fondo_anulare_continuo_canale_cavi" add sketch "Schizzo27" along normal blind 3 bodies 4 in component "01_Tetto_elettronica_removibile"
sketch "Schizzo28" plane through (0, 0, 20) normal (0, 0, 1) x (1, 0, 0) in component "01_Tetto_elettronica_removibile"
  line L0 (19.0919, 14.1421) -> (25.4558, 20.5061)
  line L1 (25.4558, 20.5061) -> (20.5061, 25.4558)
  line L2 (20.5061, 25.4558) -> (14.1421, 19.0919)
  line L3 (14.1421, 19.0919) -> (19.0919, 14.1421)
extrude "Uscita_fissa_9x7_canale_cavi_verso_vano_elettronica" cut sketch "Schizzo28" along normal blind 3 bodies 4 in component "01_Tetto_elettronica_removibile"
ref_plane "Piano di lavoro7" through (0, 0, 18) normal (0, 0, 1) x (1, 0, 0) in component "01_Tetto_elettronica_removibile"
sketch "Schizzo29" plane through (0, 0, 18) normal (0, 0, 1) x (1, 0, 0) in component "01_Tetto_elettronica_removibile"
  line L0 (23, 26) -> (41, 26)
  line L1 (41, 26) -> (41, 38)
  line L2 (41, 38) -> (23, 38)
  line L3 (23, 38) -> (23, 26)
extrude "Estrusione_Piastrina_fermacavo_fissa_sotto_uscita" add sketch "Schizzo29" along normal blind 2.2 bodies 4 in component "01_Tetto_elettronica_removibile"
sketch "Schizzo30" plane through (0, 0, 18) normal (0, 0, 1) x (1, 0, 0) in component "01_Tetto_elettronica_removibile"
  line L0 (7, 29) -> (27, 29)
  line L1 (27, 29) -> (27, 33)
  line L2 (27, 33) -> (7, 33)
  line L3 (7, 33) -> (7, 29)
extrude "Estrusione_Ponte_strutturale_fermacavo_fisso" add sketch "Schizzo30" along normal blind 2.2 bodies 4 in component "01_Tetto_elettronica_removibile"
sketch "Schizzo31" plane through (0, 0, 18) normal (0, 0, 1) x (1, 0, 0) in component "01_Tetto_elettronica_removibile"
  line L0 (31, 27.5) -> (36, 27.5)
  line L1 (36, 27.5) -> (36, 29.5)
  line L2 (36, 29.5) -> (31, 29.5)
  line L3 (31, 29.5) -> (31, 27.5)
extrude "Asola_fermacavo_fissa_inferiore_01" cut sketch "Schizzo31" along normal blind 2.2 bodies 4 in component "01_Tetto_elettronica_removibile"
sketch "Schizzo32" plane through (0, 0, 18) normal (0, 0, 1) x (1, 0, 0) in component "01_Tetto_elettronica_removibile"
  line L0 (31, 34.5) -> (36, 34.5)
  line L1 (36, 34.5) -> (36, 36.5)
  line L2 (36, 36.5) -> (31, 36.5)
  line L3 (31, 36.5) -> (31, 34.5)
extrude "Asola_fermacavo_fissa_inferiore_02" cut sketch "Schizzo32" along normal blind 2.2 bodies 4 in component "01_Tetto_elettronica_removibile"
sketch "Schizzo33" plane through (0, 0, 30) normal (0, 0, 1) x (1, 0, 0) in component "01_Tetto_elettronica_removibile"
  circle A0 centre (0, 0) radius 32.5
  circle A1 centre (0, 0) radius 23.5
extrude "Guida_anulare_cavi_azimut_meno180_piu180" cut sketch "Schizzo33" along normal blind 3 bodies 4 in component "01_Tetto_elettronica_removibile"
ref_plane "Piano di lavoro8" through (0, 0, 32.7) normal (0, 0, 1) x (1, 0, 0) in component "01_Tetto_elettronica_removibile"
sketch "Schizzo34" plane through (0, 0, 32.7) normal (0, 0, 1) x (1, 0, 0) in component "01_Tetto_elettronica_removibile"
  circle A0 centre (0, 0) radius 47.2
  circle A1 centre (0, 0) radius 37.8
extrude "Sede_ribassata_rondella_assiale" cut sketch "Schizzo34" along normal blind 0.3 bodies 4 in component "01_Tetto_elettronica_removibile"
ref_plane "Piano di lavoro9" through (0, 0, 32.5) normal (0, 0, 1) x (1, 0, 0) in component "01_Tetto_elettronica_removibile"
sketch "Schizzo35" plane through (0, 0, 32.5) normal (0, 0, 1) x (1, 0, 0) in component "01_Tetto_elettronica_removibile"
  circle A0 centre (0, 0) radius 36.5
  circle A1 centre (0, 0) radius 34.5
extrude "Estrusione_Labbro_fisso_centraggio_radiale_torretta" add sketch "Schizzo35" along normal blind 3.1 separate body makes body 5 in component "01_Tetto_elettronica_removibile"
combine "Unione_labbro_fisso_al_tetto" operation add target body 4 tool bodies 5 in component "01_Tetto_elettronica_removibile"
ref_plane "Piano di lavoro10" through (0, 0, 32.8) normal (0, 0, 1) x (1, 0, 0) in component "01_Tetto_elettronica_removibile"
sketch "Schizzo36" plane through (0, 0, 32.8) normal (0, 0, 1) x (1, 0, 0) in component "01_Tetto_elettronica_removibile"
  line L0 (51.5, -7.3) -> (61.5, -7.3)
  line L1 (61.5, -7.3) -> (61.5, -5.3)
  line L2 (61.5, -5.3) -> (51.5, -5.3)
  line L3 (51.5, -5.3) -> (51.5, -7.3)
extrude "Estrusione_Spallamento_antirotazione_Est_01" add sketch "Schizzo36" along normal blind 1.7 bodies 4 in component "01_Tetto_elettronica_removibile"
sketch "Schizzo37" plane through (0, 0, 32.8) normal (0, 0, 1) x (1, 0, 0) in component "01_Tetto_elettronica_removibile"
  line L0 (51.5, 5.3) -> (61.5, 5.3)
  line L1 (61.5, 5.3) -> (61.5, 7.3)
  line L2 (61.5, 7.3) -> (51.5, 7.3)
  line L3 (51.5, 7.3) -> (51.5, 5.3)
extrude "Estrusione_Spallamento_antirotazione_Est_02" add sketch "Schizzo37" along normal blind 1.7 bodies 4 in component "01_Tetto_elettronica_removibile"
sketch "Schizzo38" plane through (0, 0, 32.8) normal (0, 0, 1) x (1, 0, 0) in component "01_Tetto_elettronica_removibile"
  line L0 (-61.5, -7.3) -> (-51.5, -7.3)
  line L1 (-51.5, -7.3) -> (-51.5, -5.3)
  line L2 (-51.5, -5.3) -> (-61.5, -5.3)
  line L3 (-61.5, -5.3) -> (-61.5, -7.3)
extrude "Estrusione_Spallamento_antirotazione_Ovest_01" add sketch "Schizzo38" along normal blind 1.7 bodies 4 in component "01_Tetto_elettronica_removibile"
sketch "Schizzo39" plane through (0, 0, 32.8) normal (0, 0, 1) x (1, 0, 0) in component "01_Tetto_elettronica_removibile"
  line L0 (-61.5, 5.3) -> (-51.5, 5.3)
  line L1 (-51.5, 5.3) -> (-51.5, 7.3)
  line L2 (-51.5, 7.3) -> (-61.5, 7.3)
  line L3 (-61.5, 7.3) -> (-61.5, 5.3)
extrude "Estrusione_Spallamento_antirotazione_Ovest_02" add sketch "Schizzo39" along normal blind 1.7 bodies 4 in component "01_Tetto_elettronica_removibile"
sketch "Schizzo40" plane through (0, 0, 32.8) normal (0, 0, 1) x (1, 0, 0) in component "01_Tetto_elettronica_removibile"
  line L0 (-7.3, 51.5) -> (-5.3, 51.5)
  line L1 (-5.3, 51.5) -> (-5.3, 61.5)
  line L2 (-5.3, 61.5) -> (-7.3, 61.5)
  line L3 (-7.3, 61.5) -> (-7.3, 51.5)
extrude "Estrusione_Spallamento_antirotazione_Nord_01" add sketch "Schizzo40" along normal blind 1.7 bodies 4 in component "01_Tetto_elettronica_removibile"
sketch "Schizzo41" plane through (0, 0, 32.8) normal (0, 0, 1) x (1, 0, 0) in component "01_Tetto_elettronica_removibile"
  line L0 (5.3, 51.5) -> (7.3, 51.5)
  line L1 (7.3, 51.5) -> (7.3, 61.5)
  line L2 (7.3, 61.5) -> (5.3, 61.5)
  line L3 (5.3, 61.5) -> (5.3, 51.5)
extrude "Estrusione_Spallamento_antirotazione_Nord_02" add sketch "Schizzo41" along normal blind 1.7 bodies 4 in component "01_Tetto_elettronica_removibile"
sketch "Schizzo42" plane through (0, 0, 32.8) normal (0, 0, 1) x (1, 0, 0) in component "01_Tetto_elettronica_removibile"
  line L0 (-7.3, -61.5) -> (-5.3, -61.5)
  line L1 (-5.3, -61.5) -> (-5.3, -51.5)
  line L2 (-5.3, -51.5) -> (-7.3, -51.5)
  line L3 (-7.3, -51.5) -> (-7.3, -61.5)
extrude "Estrusione_Spallamento_antirotazione_Sud_01" add sketch "Schizzo42" along normal blind 1.7 bodies 4 in component "01_Tetto_elettronica_removibile"
sketch "Schizzo43" plane through (0, 0, 32.8) normal (0, 0, 1) x (1, 0, 0) in component "01_Tetto_elettronica_removibile"
  line L0 (5.3, -61.5) -> (7.3, -61.5)
  line L1 (7.3, -61.5) -> (7.3, -51.5)
  line L2 (7.3, -51.5) -> (5.3, -51.5)
  line L3 (5.3, -51.5) -> (5.3, -61.5)
extrude "Estrusione_Spallamento_antirotazione_Sud_02" add sketch "Schizzo43" along normal blind 1.7 bodies 4 in component "01_Tetto_elettronica_removibile"
ref_plane "Piano di lavoro1" through (0, 0, 32.7) normal (0, 0, 1) x (1, 0, 0) in component "02A_Rondella_assiale_torretta_sostituibile"
sketch "Schizzo1 (6)" plane through (0, 0, 32.7) normal (0, 0, 1) x (1, 0, 0) in component "02A_Rondella_assiale_torretta_sostituibile"
  circle A0 centre (0, 0) radius 47
  circle A1 centre (0, 0) radius 38
extrude "Estrusione_Rondella_assiale_basso_attrito" add sketch "Schizzo1 (6)" along normal blind 0.8 separate body makes body 6 in component "02A_Rondella_assiale_torretta_sostituibile"
ref_plane "Piano di lavoro1" through (0, 0, 10) normal (0, 0, 1) x (1, 0, 0) in component "02_Stepper_28BYJ48_statore_fisso_riferimento"
sketch "Schizzo1 (7)" plane through (0, 0, 10) normal (0, 0, 1) x (1, 0, 0) in component "02_Stepper_28BYJ48_statore_fisso_riferimento"
  circle A0 centre (0, 0) radius 14
extrude "Estrusione_Corpo_stepper" add sketch "Schizzo1 (7)" along normal blind 20 separate body makes body 7 in component "02_Stepper_28BYJ48_statore_fisso_riferimento"
ref_plane "Piano di lavoro2" through (0, 0, 27) normal (0, 0, 1) x (1, 0, 0) in component "02_Stepper_28BYJ48_statore_fisso_riferimento"
sketch "Schizzo2 (5)" plane through (0, 0, 27) normal (0, 0, 1) x (1, 0, 0) in component "02_Stepper_28BYJ48_statore_fisso_riferimento"
  line L0 (-20.75, -4) -> (20.75, -4)
  line L1 (20.75, -4) -> (20.75, 4)
  line L2 (20.75, 4) -> (-20.75, 4)
  line L3 (-20.75, 4) -> (-20.75, -4)
extrude "Estrusione_Alette_fissaggio_stepper" add sketch "Schizzo2 (5)" along normal blind 3 bodies 7 in component "02_Stepper_28BYJ48_statore_fisso_riferimento"
ref_plane "Piano di lavoro1" through (0, 0, 30) normal (0, 0, 1) x (1, 0, 0) in component "02B_Rotore_albero_28BYJ48_riferimento"
sketch "Schizzo1 (8)" plane through (0, 0, 30) normal (0, 0, 1) x (1, 0, 0) in component "02B_Rotore_albero_28BYJ48_riferimento"
  circle A0 centre (0, 0) radius 2.5
extrude "Estrusione_Albero_stepper" add sketch "Schizzo1 (8)" along normal blind 9 separate body makes body 8 in component "02B_Rotore_albero_28BYJ48_riferimento"
sketch "Schizzo2 (6)" plane through (0, 0, 30) normal (0, 0, 1) x (1, 0, 0) in component "02B_Rotore_albero_28BYJ48_riferimento"
  line L0 (-2.5, -2.7) -> (-0.5, -2.7)
  line L1 (-0.5, -2.7) -> (-0.5, 2.7)
  line L2 (-0.5, 2.7) -> (-2.5, 2.7)
  line L3 (-2.5, 2.7) -> (-2.5, -2.7)
extrude "Piatto_albero_stepper_quota_3mm" cut sketch "Schizzo2 (6)" along normal blind 9 bodies 8 in component "02B_Rotore_albero_28BYJ48_riferimento"
ref_plane "Piano di lavoro1" through (0, 0, 33.5) normal (0, 0, 1) x (1, 0, 0) in component "03_Base_rotante_D100_sede_D_stepper"
sketch "Schizzo1 (9)" plane through (0, 0, 33.5) normal (0, 0, 1) x (1, 0, 0) in component "03_Base_rotante_D100_sede_D_stepper"
  circle A0 centre (0, 0) radius 50
extrude "Estrusione_Piastra_base_rotante_D100" add sketch "Schizzo1 (9)" along normal blind 6 separate body makes body 9 in component "03_Base_rotante_D100_sede_D_stepper"
sketch "Schizzo2 (7)" plane through (0, 0, 33.5) normal (0, 0, 1) x (1, 0, 0) in component "03_Base_rotante_D100_sede_D_stepper"
  circle A0 centre (0, 0) radius 2.7
extrude "Preforo_circolare_sede_D_stepper" cut sketch "Schizzo2 (7)" along normal blind 6 bodies 8 in component "02B_Rotore_albero_28BYJ48_riferimento"
extrude "Estrusione2" cut sketch "Schizzo2 (7)" along normal blind 6 bodies 9 in component "03_Base_rotante_D100_sede_D_stepper"
sketch "Schizzo3 (5)" plane through (0, 0, 33.5) normal (0, 0, 1) x (1, 0, 0) in component "03_Base_rotante_D100_sede_D_stepper"
  line L0 (-2.7, -2.9) -> (-0.5, -2.9)
  line L1 (-0.5, -2.9) -> (-0.5, 2.9)
  line L2 (-0.5, 2.9) -> (-2.7, 2.9)
  line L3 (-2.7, 2.9) -> (-2.7, -2.9)
extrude "Estrusione_Riempimento_lato_piatto_sede_D" add sketch "Schizzo3 (5)" along normal blind 6 bodies 9 in component "03_Base_rotante_D100_sede_D_stepper"
sketch "Schizzo4 (5)" plane through (0, 0, 33.5) normal (0, 0, 1) x (1, 0, 0) in component "03_Base_rotante_D100_sede_D_stepper"
  circle A0 centre (0, 0) radius 36.8
  circle A1 centre (0, 0) radius 34.2
extrude "Gola_inferiore_centraggio_radiale_con_gioco" cut sketch "Schizzo4 (5)" along normal blind 2.5 bodies 4 in component "01_Tetto_elettronica_removibile"
extrude "Estrusione4" cut sketch "Schizzo4 (5)" along normal blind 2.5 bodies 9 in component "03_Base_rotante_D100_sede_D_stepper"
ref_plane "Piano di lavoro2" through (0, 0, 36.9) normal (0, 0, 1) x (1, 0, 0) in component "03_Base_rotante_D100_sede_D_stepper"
sketch "Schizzo5 (5)" plane through (0, 0, 33.5) normal (0, 0, 1) x (1, 0, 0) in component "03_Base_rotante_D100_sede_D_stepper"
  circle A0 centre (-19, 0) radius 1.6
extrude "Foro_M3_adattatore_01" cut sketch "Schizzo5 (5)" along normal blind 6 bodies 9 in component "03_Base_rotante_D100_sede_D_stepper"
sketch "Schizzo6 (5)" plane through (0, 0, 36.9) normal (0, 0, 1) x (1, 0, 0) in component "03_Base_rotante_D100_sede_D_stepper"
  line L0 (-16.1, 1.6743) -> (-19, 3.3486)
  line L1 (-19, 3.3486) -> (-21.9, 1.6743)
  line L2 (-21.9, 1.6743) -> (-21.9, -1.6743)
  line L3 (-21.9, -1.6743) -> (-19, -3.3486)
  line L4 (-19, -3.3486) -> (-16.1, -1.6743)
  line L5 (-16.1, -1.6743) -> (-16.1, 1.6743)
extrude "Sede_dado_M3_adattatore_01" cut sketch "Schizzo6 (5)" along normal blind 2.6 bodies 9 in component "03_Base_rotante_D100_sede_D_stepper"
sketch "Schizzo7 (5)" plane through (0, 0, 33.5) normal (0, 0, 1) x (1, 0, 0) in component "03_Base_rotante_D100_sede_D_stepper"
  circle A0 centre (19, 0) radius 1.6
extrude "Foro_M3_adattatore_02" cut sketch "Schizzo7 (5)" along normal blind 6 bodies 9 in component "03_Base_rotante_D100_sede_D_stepper"
sketch "Schizzo8 (5)" plane through (0, 0, 36.9) normal (0, 0, 1) x (1, 0, 0) in component "03_Base_rotante_D100_sede_D_stepper"
  line L0 (21.9, 1.6743) -> (19, 3.3486)
  line L1 (19, 3.3486) -> (16.1, 1.6743)
  line L2 (16.1, 1.6743) -> (16.1, -1.6743)
  line L3 (16.1, -1.6743) -> (19, -3.3486)
  line L4 (19, -3.3486) -> (21.9, -1.6743)
  line L5 (21.9, -1.6743) -> (21.9, 1.6743)
extrude "Sede_dado_M3_adattatore_02" cut sketch "Schizzo8 (5)" along normal blind 2.6 bodies 9 in component "03_Base_rotante_D100_sede_D_stepper"
sketch "Schizzo9 (5)" plane through (0, 0, 33.5) normal (0, 0, 1) x (1, 0, 0) in component "03_Base_rotante_D100_sede_D_stepper"
  circle A0 centre (0, -19) radius 1.6
extrude "Foro_M3_adattatore_03" cut sketch "Schizzo9 (5)" along normal blind 6 bodies 9 in component "03_Base_rotante_D100_sede_D_stepper"
sketch "Schizzo10 (5)" plane through (0, 0, 36.9) normal (0, 0, 1) x (1, 0, 0) in component "03_Base_rotante_D100_sede_D_stepper"
  line L0 (2.9, -17.3257) -> (0, -15.6514)
  line L1 (0, -15.6514) -> (-2.9, -17.3257)
  line L2 (-2.9, -17.3257) -> (-2.9, -20.6743)
  line L3 (-2.9, -20.6743) -> (0, -22.3486)
  line L4 (0, -22.3486) -> (2.9, -20.6743)
  line L5 (2.9, -20.6743) -> (2.9, -17.3257)
extrude "Sede_dado_M3_adattatore_03" cut sketch "Schizzo10 (5)" along normal blind 2.6 bodies 9 in component "03_Base_rotante_D100_sede_D_stepper"
sketch "Schizzo11 (5)" plane through (0, 0, 33.5) normal (0, 0, 1) x (1, 0, 0) in component "03_Base_rotante_D100_sede_D_stepper"
  circle A0 centre (0, 19) radius 1.6
extrude "Foro_M3_adattatore_04" cut sketch "Schizzo11 (5)" along normal blind 6 bodies 9 in component "03_Base_rotante_D100_sede_D_stepper"
sketch "Schizzo12 (4)" plane through (0, 0, 36.9) normal (0, 0, 1) x (1, 0, 0) in component "03_Base_rotante_D100_sede_D_stepper"
  line L0 (2.9, 20.6743) -> (0, 22.3486)
  line L1 (0, 22.3486) -> (-2.9, 20.6743)
  line L2 (-2.9, 20.6743) -> (-2.9, 17.3257)
  line L3 (-2.9, 17.3257) -> (0, 15.6514)
  line L4 (0, 15.6514) -> (2.9, 17.3257)
  line L5 (2.9, 17.3257) -> (2.9, 20.6743)
extrude "Sede_dado_M3_adattatore_04" cut sketch "Schizzo12 (4)" along normal blind 2.6 bodies 9 in component "03_Base_rotante_D100_sede_D_stepper"
sketch "Schizzo13 (4)" plane through (0, 0, 33.5) normal (0, 0, 1) x (1, 0, 0) in component "03_Base_rotante_D100_sede_D_stepper"
  line L0 (19.0919, 14.1421) -> (25.4558, 20.5061)
  line L1 (25.4558, 20.5061) -> (20.5061, 25.4558)
  line L2 (20.5061, 25.4558) -> (14.1421, 19.0919)
  line L3 (14.1421, 19.0919) -> (19.0919, 14.1421)
extrude "Passaggio_9x7_comune_servi_cannone_adattatore" cut sketch "Schizzo13 (4)" along normal blind 6 bodies 9 in component "03_Base_rotante_D100_sede_D_stepper"
ref_plane "Piano di lavoro1" through (0, 0, 33) normal (0, 0, 1) x (1, 0, 0) in component "03A_Fermaglio_anti_sollevamento_Est_M3"
ref_plane "Piano di lavoro2" through (0, 0, 36) normal (0, 0, 1) x (1, 0, 0) in component "03A_Fermaglio_anti_sollevamento_Est_M3"
ref_plane "Piano di lavoro3" through (0, 0, 39.9) normal (0, 0, 1) x (1, 0, 0) in component "03A_Fermaglio_anti_sollevamento_Est_M3"
sketch "Schizzo1 (10)" plane through (0, 0, 33) normal (0, 0, 1) x (1, 0, 0) in component "03A_Fermaglio_anti_sollevamento_Est_M3"
  line L0 (51.5, -5) -> (61.5, -5)
  line L1 (61.5, -5) -> (61.5, 5)
  line L2 (61.5, 5) -> (51.5, 5)
  line L3 (51.5, 5) -> (51.5, -5)
extrude "Estrusione_Piede_fermaglio_Est" add sketch "Schizzo1 (10)" along normal blind 3 separate body makes body 10 in component "03A_Fermaglio_anti_sollevamento_Est_M3"